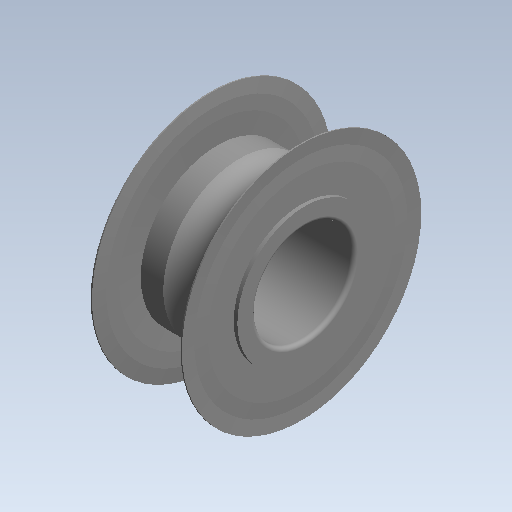
# Autodesk Inventor part: W 605-2Z_PART1
Saved by Autodesk Inventor 2020.2 (Build 242310000, 310)
## iProperties
Part Number: W 605-2Z_PART1
Material: Generic
Catalog Web Link: www.cadenas.de
Description: -Deep groove ball bearings
Vendor: SKF
Document SubType Name: Modeling
Designer: partserver
Manufacturer: SKF
Mass: 0.134836 g
Surface Area: 5.69453 cm^2
Volume: 0.134836 cm^3
Density: 1 g/cm^3
Appearance: PSOLRGB-175-175-175
Category: PARTsolutions
Company: SKF
PSOL_IDENT_0: {$CADENAS_DATA\23d-libs\skf\bearings_units_and_housings\ball_bearings\deep_groove_ball_bearings\bb1_
PSOL_IDENT_1: 001_101.prj},195 {VTYP=3D},{NB=W 605-2Z_PART1},{LINA=W 605-2Z_PART1},{NN=BB1_001_101_PART1},{NOPRJ=T
PSOL_IDENT_2: RUE},{DATE=26.02.2021 12:30:54},{GEOMDATE=05.02.2021 06:24:08},{VERSION=},{LINEID=16160},{WBVAR=},{W
PSOL_IDENT_3: BNUMERIC=}  {NB=W 605-2Z_PART1},{LINA=W 605-2Z_PART1},{KT=DUMMY},{DESIGNATION=W 605-2Z},{R12=0.20},{
PSOL_IDENT_4: DD=5.000},{D=14.000},{B=5.000},{C=},{CX=},{CXX=},{CA=0.000},{XXVARIANT=},{XXDESIGN=Single row stainl
PSOL_IDENT_5: ess steel},{XXSEALING=Shield on both sides},{DESIGN=dgbbw2z},{DESIGNIR=dgbbw2z},{VARIANT=},{DD1=7.79
PSOL_IDENT_6: },{DD2=6.9},{DD2X=},{DD2A=6.90},{D1=11.28},{D1X=MIN},{D2=12.2},{D2A=12.20},{D3=},{D3X=},{D3A=0.000},
PSOL_IDENT_7: {D4=},{HH=MIN},{BB=0.000},{BBX=},{BBA=0.000},{FF=},{R0MAX=MIN},{R0=MIN},{PITCH=9.50},{DW=2.381},{DDA
PSOL_IDENT_8: MIN=6.600},{DDAMAX=6.800},{DDBMIN=MIN},{DDBMAX=MIN},{DBMIN=MIN},{DAMAX=12.400},{BBAMIN=MIN},{CAMAX=M
PSOL_IDENT_9: IN},{RAMAX=0.200},{LOAD1=0.761},{LOAD2=0.260},{LOAD3=0.011},{SPEED1=110000},{SPEED2=53000},{KR=0.030
PSOL_IDENT_10: },{F0=6.600},{Z=7},{II=1},{MASS=0.003},{BEARING=W 605-2Z},{RING=},{HELP=1.360},{HELP2=0.900},{DD1ALG=
PSOL_IDENT_11: 3.895},{YALG=3.895},{PITCH1=9.500},{DW1=2.381},{YALG1=5.640},{HALG1=1.360},{SH=3.450},{CU=0.524},{HA
PSOL_IDENT_12: LG=1.395},{B1=0},{SHIELDHELP=2},{D4A=0.000},{FFA=0.000},{RS1=}
NB: W 605-2Z_PART1
NT: Deep groove ball bearings
NBSYN: $DESIGNATION._PART1
LINA: W 605-2Z_PART1
CATALOG: SKF
SUPPLIER: SKF
ARTICLENO: W 605-2Z_PART1
BOMINFO: W 605-2Z_PART1
CREATOR: CADENAS GmbH
Title: W 605-2Z_PART1
Author: Cadenas PARTsolutions
Comments: Deep groove ball bearings
Autodesk Inventor part; units mm, degrees
ref_plane "YZ Plane" through (0, 0, 0) normal (1, 0, 0) x (0, 1, 0)
ref_plane "XZ Plane" through (0, 0, 0) normal (0, 1, 0) x (-1, 0, 0)
ref_plane "XY Plane" through (0, 0, 0) normal (0, 0, 1) x (1, 0, 0)
sketch "Sketch_17" plane through (0, 0, 0) normal (0, 0, 1) x (1, 0, 0)
  line L0 (50, 0) -> (-50, 0)
  line L1 (0, 3.855) -> (0, 2.7)
  arc A0 (0, 2.7) -> (0.2, 2.5) centre (0.2, 2.7) ccw
  line L2 (0.2, 2.5) -> (4.8, 2.5)
  arc A1 (4.8, 2.5) -> (5, 2.7) centre (4.8, 2.7) ccw
  line L3 (5, 2.7) -> (5, 3.855)
  arc A2 (5, 3.855) -> (4.96, 3.895) centre (4.96, 3.855) ccw
  line L4 (4.96, 3.895) -> (3.3284, 3.895)
  arc A3 (1.6716, 3.895) -> (3.3284, 3.895) centre (2.5, 4.75) ccw
  line L5 (1.6716, 3.895) -> (0.04, 3.895)
  arc A4 (0.04, 3.895) -> (0, 3.855) centre (0.04, 3.855) ccw
  constraints: 12 end point, 10 point on circle, 5 centre point
revolve "Revolution1" add sketch "Sketch_17" angle 360 about axis through (50, 0, 0) along (1, 0, 0)
sketch "Sketch_19" plane through (0, 0, 0) normal (0, 0, 1) x (1, 0, 0)
  line L0 (50, 0) -> (-50, 0)
  line L1 (0, 4.6375) -> (0, 3.45)
  line L2 (0, 3.45) -> (0.3057, 3.45)
  arc A0 (0.3057, 3.45) -> (0.524, 3.6683) centre (0.3057, 3.6683) ccw
  line L3 (0.524, 3.6683) -> (0.524, 4.2882)
  line L4 (0.524, 4.2882) -> (4.476, 4.2882)
  line L5 (4.476, 4.2882) -> (4.476, 3.6683)
  arc A1 (4.476, 3.6683) -> (4.6943, 3.45) centre (4.6943, 3.6683) ccw
  line L6 (4.6943, 3.45) -> (5, 3.45)
  line L7 (5, 3.45) -> (5, 4.6375)
  line L8 (5, 4.6375) -> (0, 4.6375)
  constraints: 18 end point, 4 point on circle, 2 centre point
revolve "Revolution2" cut sketch "Sketch_19" angle 360 about axis through (50, 0, 0) along (1, 0, 0)
sketch "Sketch_20" plane through (0, 0, 0) normal (0, 0, 1) x (1, 0, 0)
  line L0 (50, 0) -> (-50, 0)
  line L1 (0.18, 6.1) -> (0.21, 5.435)
  line L2 (0.21, 5.435) -> (0.18, 4.77)
  line L3 (0.18, 4.77) -> (0.18, 3.44)
  line L4 (0.18, 3.44) -> (0.24, 3.44)
  line L5 (0.24, 3.44) -> (0.3, 4.77)
  line L6 (0.3, 4.77) -> (0.3, 5.435)
  line L7 (0.3, 5.435) -> (0.24, 6.1)
  line L8 (0.24, 6.1) -> (0.18, 6.1)
  constraints: 18 end point
revolve "Revolution3" add sketch "Sketch_20" angle 360 about axis through (50, 0, 0) along (1, 0, 0)
sketch "Sketch_21" plane through (0, 0, 0) normal (0, 0, 1) x (1, 0, 0)
  line L0 (50, 0) -> (-50, 0)
  line L1 (4.7, 5.435) -> (4.7, 4.77)
  line L2 (4.7, 4.77) -> (4.76, 3.44)
  line L3 (4.76, 3.44) -> (4.82, 3.44)
  line L4 (4.82, 3.44) -> (4.82, 4.77)
  line L5 (4.82, 4.77) -> (4.79, 5.435)
  line L6 (4.79, 5.435) -> (4.82, 6.1)
  line L7 (4.82, 6.1) -> (4.76, 6.1)
  line L8 (4.76, 6.1) -> (4.7, 5.435)
  constraints: 18 end point
revolve "Revolution4" add sketch "Sketch_21" angle 360 about axis through (50, 0, 0) along (1, 0, 0)
body "Solid1"
